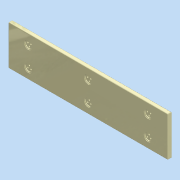
# Autodesk Inventor part: Platt oben
Saved by Autodesk Inventor 2021 (Build 250183000, 183)
## iProperties
Created: 2024-03-13
Part Number: Platt oben
Material: Generic
Document SubType Name: Modeling
Designer: Nokia
Density: 1 g/cm^3
Appearance: Smooth - Ash
Mass: 3100.69 g
Surface Area: 3710.93 cm^2
Volume: 3100.69 cm^3
Author: Nokia
Autodesk Inventor part; units mm, degrees
ref_plane "YZ Plane" through (0, 0, 0) normal (1, 0, 0) x (0, 1, 0)
ref_plane "XZ Plane" through (0, 0, 0) normal (0, 1, 0) x (-1, 0, 0)
ref_plane "XY Plane" through (0, 0, 0) normal (0, 0, 1) x (1, 0, 0)
sketch "Sketch1" plane through (0, 0, 0) normal (0, 0, 1) x (1, 0, 0)
  line L0 (-400, -100) -> (-400, 100)
  line L1 (-400, 100) -> (400, 100)
  line L2 (400, 100) -> (400, -100)
  line L3 (400, -100) -> (-400, -100)
  point P0 (0, 0)
  dimension "d2" = 800
  dimension "d3" = 200
  constraints: 8 end point, 3 perpendicular
  measures "d2" distance of L0.end L1.end
  measures "d3" distance of L1.end L2.end
extrude "Extrusion1" add sketch "Sketch1" along normal blind 20
sketch "Sketch5" plane through (0, 0, 20) normal (0, 0, 1) x (1, 0, 0)
  line L0 (0, 0) -> (0, 50)
  circle A0 centre (0, 50) radius 17
  line L1 (0, 0) -> (-150, 0)
  line L2 (-150, 0) -> (-150, 100)
  line L3 (-400, 100) -> (400, 100)
  circle A1 centre (0, -50) radius 17
  circle A2 centre (-300, 50) radius 17
  circle A3 centre (-300, -50) radius 17
  circle A4 centre (300, 50) radius 17
  circle A5 centre (300, -50) radius 17
  circle A6 centre (0, 50) radius 20
  circle A7 centre (0, -50) radius 20
  circle A8 centre (-300, 50) radius 20
  circle A9 centre (-300, -50) radius 20
  circle A10 centre (300, -50) radius 20
  circle A11 centre (300, 50) radius 20
  dimension "d18" = 50
  dimension "d19" = 34
  dimension "d20" = 150
  dimension "d43" = 40
  constraints: 12 centre point, 10 symmetric about line, 8 end point, 2 coincident, 1 horizontal, 1 perpendicular, 1 point on line, 1 vertical, 10 other
  measures "d18" distance of L0.start L0.end
  measures "d19" diameter of A0
  measures "d20" distance of L0.start L1.end
  measures "d43" diameter of A6
extrude "Extrusion4" cut sketch "Sketch5" against normal blind 6 contours A0 | A1 | A2 | A3 | A4 | A5
sketch "Sketch6" plane through (0, 0, 0) normal (0, 0, -1) x (-1, 0, 0)
  line L0 (0, 0) -> (0, 50)
  circle A0 centre (0, 50) radius 20
  line L1 (0, 0) -> (-150, 0)
  line L2 (-150, 0) -> (-150, 100)
  line L3 (-400, 100) -> (400, 100)
  circle A1 centre (0, -50) radius 20
  circle A2 centre (-300, 50) radius 20
  circle A3 centre (-300, -50) radius 20
  circle A4 centre (300, 50) radius 20
  circle A5 centre (300, -50) radius 20
  circle A6 centre (0, 50) radius 15
  circle A7 centre (9, 50) radius 3.5
  circle A8 centre (-4.5, 57.7942) radius 3.5
  circle A9 centre (-4.5, 42.2058) radius 3.5
  circle A10 centre (0, -50) radius 15
  circle A11 centre (9, -50) radius 3.5
  circle A12 centre (-4.5, -57.7942) radius 3.5
  circle A13 centre (-4.5, -42.2058) radius 3.5
  circle A14 centre (-300, 50) radius 15
  circle A15 centre (-309, 50) radius 3.5
  circle A16 centre (-295.5, 57.7942) radius 3.5
  circle A17 centre (-295.5, 42.2058) radius 3.5
  circle A18 centre (-295.5, -57.7942) radius 3.5
  circle A19 centre (-309, -50) radius 3.5
  circle A20 centre (-295.5, -42.2058) radius 3.5
  circle A21 centre (-300, -50) radius 15
  circle A22 centre (300, -50) radius 15
  circle A23 centre (295.5, -42.2058) radius 3.5
  circle A24 centre (309, -50) radius 3.5
  circle A25 centre (295.5, -57.7942) radius 3.5
  circle A26 centre (309, 50) radius 3.5
  circle A27 centre (295.5, 42.2058) radius 3.5
  circle A28 centre (295.5, 57.7942) radius 3.5
  circle A29 centre (300, 50) radius 15
  dimension "d23" = 50
  dimension "d24" = 40
  dimension "d25" = 150
  dimension "d28" = 30
  dimension "d30" = 7
  dimension "d33" = 360
  dimension "d58" = 9
  dimension "d59" = 0
  constraints: 30 centre point, 25 symmetric about line, 8 end point, 2 coincident, 1 horizontal, 1 perpendicular, 1 point on line, 1 vertical, 33 other
  measures "d23" distance of L0.start L0.end
  measures "d24" diameter of A0
  measures "d25" distance of L0.start L1.end
  measures "d28" diameter of A6
  measures "d30" diameter of A7
  measures "d58" distance from line of L0 A7.centre
  measures "d59" vertical distance of L0.end A7.centre
extrude "Extrusion5" cut sketch "Sketch6" against normal blind 8 contours A0 | A1 | A2 | A3 | A4 | A5 | A6 | A7 | A8 | A9 | A10 | A11 | A12 | A13 | A14 | A15 | A16 | A17 | A18 | A19 | A20 | A21 | A22 | A23 | A24 | A25 | A26 | A27 | A28 | A29
hole "Hole1" at (-295.5, -57.7942, 0) at (-295.5, -42.2058, 0) at (-309, -50, 0) at (-309, 50, 0) at (-295.5, 57.7942, 0) at (-295.5, 42.2058, 0) at (4.5, -57.7942, 0) at (4.5, -42.2058, 0) at (-9, -50, 0) at (4.5, 57.7942, 0) at (-9, 50, 0) at (4.5, 42.2058, 0) at (295.5, -42.2058, 0) at (309, -50, 0) at (295.5, -57.7942, 0) at (295.5, 42.2058, 0) at (309, 50, 0) at (295.5, 57.7942, 0) direction (0, 0, 1) diameter 7 depth 55
extrude "Extrusion6" cut sketch "Sketch5" against normal blind 2
fillet "Fillet3" radius 4 11 edges at (0, -100, 0) (0, -100, 20) (400, -100, 10) (400, 0, 20) (400, 100, 10) (0, 100, 20) (0, 100, 0) (-400, -100, 10) (-400, 0, 0) (-400, 100, 10) (-400, 0, 20)
chamfer "Chamfer3" distance 1 angle 45 6 edges at (320, 50, 0) (320, -50, 0) (20, 50, 0) (20, -50, 0) (-280, 50, 0) (-280, -50, 0)
chamfer "Chamfer4" distance 0.5 angle 45 12 edges at (280, 50, 20) (283, 50, 18) (280, -50, 20) (283, -50, 18) (-20, 50, 20) (-17, 50, 18) (-17, -50, 18) (-20, -50, 20) (-320, 50, 20) (-317, 50, 18) (-320, -50, 20) (-317, -50, 18)
body "Solid1"
